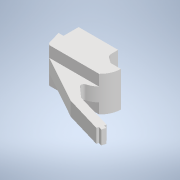
# Autodesk Inventor part: Деталь8
Saved by Autodesk Inventor 2021.2 (Build 252289000, 289)
## iProperties
Created: 2021-10-12
Part Number: Деталь8
Material: Типовые
Document SubType Name: Modeling
Designer: Surflay
Density: 1 g/cm^3
Appearance: По умолчанию
Author: Surflay
Autodesk Inventor part; units mm, degrees
ref_plane "YZ Plane" through (0, 0, 0) normal (1, 0, 0) x (0, 1, 0)
ref_plane "XZ Plane" through (0, 0, 0) normal (0, 1, 0) x (-1, 0, 0)
ref_plane "XY Plane" through (0, 0, 0) normal (0, 0, 1) x (1, 0, 0)
sketch "Эскиз1" plane through (0, 0, 0) normal (0, 0, 1) x (1, 0, 0)
  line L0 (33.5, -8.5) -> (33.5, 11.5) projected
  line L1 (28.5, 11.5) -> (-21.5, 11.5)
  line L2 (-21.5, 11.5) -> (-21.5, -8.5)
  line L3 (-21.5, -8.5) -> (28.5, -8.5)
  line L4 (28.5, -8.5) -> (28.5, 11.5)
  point P0 (0, 0)
  point P1 (28.5, 1.5)
  point P2 (33.5, 1.5)
  dimension "d0" = 20
  dimension "d1" = 50
  dimension "d2" = 5
  constraints: 8 end point, 2 midpoint, 2 parallel, 1 horizontal, 1 horizontal alignment, 1 perpendicular
  measures "d0" distance between parallel lines of L3 L1
  measures "d1" distance of L1.start L1.end
  measures "d2" distance between parallel lines of L0 L4
extrude "Выдавливание1" add sketch "Эскиз1" along normal blind 35
sketch "Эскиз2" plane through (-21.5, 11.5, 0) normal (0, 1, 0) x (1, 0, 0)
  line L0 (34.9155, -7.2898) -> (19.9439, -7.2898)
  arc A0 (29.433, -14.5026) -> (34.9155, -7.2898) centre (27.4297, -7.2898) ccw
  line L1 (29.0336, -16.2113) -> (32.723, -19.5135)
  line L2 (32.723, -19.5135) -> (45.8164, -23.3718)
  line L3 (45.8164, -23.3718) -> (45.6044, -24.0912)
  line L4 (45.6044, -24.0912) -> (46.806, -24.4452)
  line L5 (46.806, -24.4452) -> (46.382, -25.8841)
  line L6 (46.382, -25.8841) -> (45.1805, -25.53)
  line L7 (45.1805, -25.53) -> (44.9685, -26.2494)
  line L8 (44.9685, -26.2494) -> (31.875, -22.3912)
  line L9 (31.875, -22.3912) -> (21.5, -16.6598)
  line L10 (21.5, -16.6598) -> (19.9439, -14.1649)
  line L11 (19.9439, -14.1649) -> (19.9439, -7.2898)
  line L12 (31.8727, -7.2898) -> (27.4716, -4.0907)
  line L13 (26.6475, -2.4729) -> (26.6475, 0)
  line L14 (0, 0) -> (50, 0) projected
  line L15 (12.3278, 0) -> (12.3278, -7.1542)
  line L16 (12.3278, -7.1542) -> (13.5221, -11.5576)
  line L17 (14.4853, -12.7847) -> (21.5, -16.6598)
  arc A1 (29.433, -14.5026) -> (29.0336, -16.2113) centre (29.7006, -15.4662) ccw
  arc A2 (13.5221, -11.5576) -> (14.4853, -12.7847) centre (15.4524, -11.0341) ccw
  arc A3 (26.6475, -2.4729) -> (27.4716, -4.0907) centre (28.6475, -2.4729) ccw
  point P0 (21.5, 0)
  point P1 (27.4297, -14.7757)
  point P2 (13.7439, -12.3751)
  dimension "d5" = 1
  dimension "d6" = 2
  dimension "d7" = 0.75
  dimension "d8" = 3
  dimension "d9" = 1.5
  constraints: 34 end point, 9 point on circle, 7 point on line, 6 tangent, 4 centre point, 3 perpendicular, 3 vertical, 2 parallel, 1 collinear, 1 equal radius, 1 horizontal, 1 midpoint
  measures "d5" radius of A1
  measures "d6" radius of A2
  measures "d7" distance between parallel lines of L6 L8
  measures "d8" distance between parallel lines of L8 L2
  measures "d9" distance between parallel lines of L6 L4
extrude "Выдавливание2" cut sketch "Эскиз2" against normal through all keep common part
sketch "Эскиз3" plane through (-9.1722, 11.5, 0) normal (-1, 0, 0) x (0, 0, 1)
  line L0 (26.2494, 0) -> (26.2494, -20) projected
  line L1 (12.7847, 0) -> (12.7847, -20) projected
  line L2 (26.2494, -7.5889) -> (12.7847, -7.5889)
  line L3 (12.7847, -7.5889) -> (12.7847, -12.5875)
  line L4 (12.7847, -12.5875) -> (26.2494, -12.5875)
  line L5 (26.2494, -12.5875) -> (26.2494, -7.5889)
  line L6 (7.2898, 0) -> (7.2898, -20) projected
  line L7 (12.7847, -3.5953) -> (7.2898, -3.5953)
  line L8 (7.2898, -3.5953) -> (7.2898, -16.3417)
  line L9 (7.2898, -16.3417) -> (12.7847, -16.3417)
  line L10 (12.7847, -16.3417) -> (12.7847, -3.5953)
  line L11 (0, -20) -> (0, 0) projected
  line L12 (7.2898, -5.3948) -> (0, -5.3948)
  line L13 (0, -5.3948) -> (0, -14.7921)
  line L14 (0, -14.7921) -> (7.2898, -14.7921)
  line L15 (7.2898, -14.7921) -> (7.2898, -5.3948)
  point P0 (0, -11.5)
  point P1 (12.7847, -7.5889)
  point P2 (7.2898, -3.5953)
  point P3 (7.2898, -5.3948)
  point P4 (0, -5.3948)
  constraints: 24 end point, 6 parallel, 6 point on line, 3 horizontal, 3 perpendicular
extrude "Выдавливание3" cut sketch "Эскиз3" against normal blind 35 keep common part
